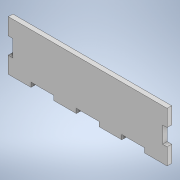
# Autodesk Inventor part: back
Saved by Autodesk Inventor 2020 (Build 240168000, 168)
## iProperties
Created: 2020-02-22
Part Number: back
Material: Generic
Document SubType Name: Modeling
Designer: udvarhelyi
Density: 1 g/cm^3
Appearance: Default
Author: udvarhelyi
Autodesk Inventor part; units mm, degrees
ref_plane "YZ Plane" through (0, 0, 0) normal (1, 0, 0) x (0, 1, 0)
ref_plane "XZ Plane" through (0, 0, 0) normal (0, 1, 0) x (-1, 0, 0)
ref_plane "XY Plane" through (0, 0, 0) normal (0, 0, 1) x (1, 0, 0)
sketch "Sketch1" plane through (0, 0, 0) normal (0, 0, 1) x (1, 0, 0)
  line L0 (-22.5, 0) -> (-22.5, 3)
  line L1 (-22.5, 3) -> (-37.5, 3)
  line L2 (-37.5, 3) -> (-37.5, 0)
  line L3 (7.5, 0) -> (7.5, 3)
  line L4 (7.5, 3) -> (-7.5, 3)
  line L5 (-7.5, 3) -> (-7.5, 0)
  line L6 (37.5, 0) -> (37.5, 3)
  line L7 (37.5, 3) -> (22.5, 3)
  line L8 (22.5, 3) -> (22.5, 0)
  line L9 (-52.5, 22) -> (-49.5, 22)
  line L10 (-49.5, 22) -> (-49.5, 11)
  line L11 (-49.5, 11) -> (-52.5, 11)
  line L12 (52.5, 11) -> (49.5, 11)
  line L13 (49.5, 11) -> (49.5, 22)
  line L14 (49.5, 22) -> (52.5, 22)
  line L15 (-37.5, 33) -> (-52.5, 33)
  line L16 (52.5, 33) -> (56.4286, 33)
  line L17 (22.5, 33) -> (2.4524, 33)
  line L18 (-7.5, 33) -> (-27.5476, 33)
  line L19 (52.5, 0) -> (52.5, 11)
  line L20 (52.5, 22) -> (52.5, 33)
  line L21 (37.5, 0) -> (52.5, 0)
  line L22 (7.5, 0) -> (22.5, 0)
  line L23 (-52.5, 0) -> (-37.5, 0)
  line L24 (-22.5, 0) -> (-7.5, 0)
  line L25 (-52.5, 33) -> (-52.5, 22)
  line L26 (-52.5, 11) -> (-52.5, 0)
  line L27 (-37.5, 33) -> (57.8569, 33)
  point P0 (0, 0)
  point P1 (0, 30)
  dimension "d46" = 105
  dimension "d48" = 33
  dimension "d49" = 52.5
  dimension "d50" = 0
  dimension "d53" = 0
  dimension "d58" = 11
  dimension "d59" = 11
  dimension "d61" = 15
  dimension "d62" = 7.5
  dimension "d63" = 3
  dimension "d64" = 3
  dimension "d65" = 3
  constraints: 56 end point, 25 parallel, 11 perpendicular, 10 collinear, 8 equal length, 8 point on line, 6 horizontal, 1 other
  measures "d46" distance of L16.start L15.end
  measures "d48" distance between parallel lines of L21 L16
  measures "d49" distance from line of L20 point (0, 0)
  measures "d50" distance from line of L21 point (0, 0)
  measures "d53" horizontal distance of point (0, 0) point (0, 30)
  measures "d58" distance of L15.end L9.start
  measures "d59" distance of L9.end L10.end
  measures "d61" distance of L0.start L5.end
  measures "d62" distance from line of L5 point (0, 0)
  measures "d63" distance of L9.start L9.end
  measures "d64" distance of L13.end L14.end
  measures "d65" distance of L1.end L2.end
extrude "Extrusion1" add sketch "Sketch1" along normal blind 3
equation "\"d46\" = shelfWs"
equation "\"d48\" = shelfD"
equation "\"d49\" = 0.5 * shelfWs"
equation "\"d58\" = 0.333333 * shelfD - tol"
equation "\"d59\" = 0.333333 * shelfD + 2 * tol"
equation "\"d24\" = tt"
equation "\"d0\" = 0.5 * shelfWs"
equation "\"tt\" = 3"
equation "\"tol\" = 0"
equation "\"d2\" = shelfD"
equation "\"d4\" = tt"
equation "\"tiroir\" = 1"
equation "\"nHoles\" = 4"
equation "\"shelfH\" = 35"
equation "\"shelfWs\" = 105"
equation "\"d47\" = 0.5 * shelfWs"
equation "\"shelfD\" = 33"
body "Solid1"
